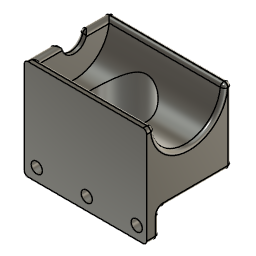
camera mount v2 (Autodesk Fusion 360 design; units mm, degrees)
Autodesk Fusion 360 part; units mm, degrees
sketch "Sketch1" plane through (0, 0, 0) normal (0, 0, 1) x (1, 0, 0)
  line L0 (0, 0) -> (49, 0)
  line L1 (49, 0) -> (49, 34)
  line L2 (49, 34) -> (0, 34)
  line L3 (0, 34) -> (0, 0)
  dimension "d1" = 49
  dimension "d2" = 34
  constraint horizontal L0
  constraint vertical L1
  constraint horizontal L2
  constraint vertical L3
  constraint coincident L0.start L3.end
  measures "d1" distance of L0.start L0.end
  measures "d2" distance of L0.start L2.end
extrude "Extrude1" add sketch "Sketch1" along normal blind 30
sketch "Sketch2" plane through (49, 0, 0) normal (1, 0, 0) x (0, 1, 0)
  line L0 (0, 0) -> (34, 0)
  line L1 (34, 0) -> (34, 30)
  line L2 (34, 30) -> (0, 30)
  line L3 (0, 30) -> (0, 0)
  circle A0 centre (17, 30) radius 14
  dimension "d5" = 28
  constraint midpoint L2 A0.centre
  measures "d5" diameter of A0
extrude "Extrude2" cut sketch "Sketch2" against normal blind 46 contours L2 A0 picked at (19.9096, 26.3515)
sketch "Sketch3" plane through (0, 0, 0) normal (0, 0, 1) x (1, 0, 0)
  circle A0 centre (21, 17) radius 11
  dimension "d10" = 22
  measures "d10" diameter of A0
extrude "Extrude3" cut sketch "Sketch3" along normal blind 40
sketch "Sketch4" plane through (3, 0, 0) normal (1, 0, 0) x (0, 1, 0)
  line L0 (31, 30) -> (3, 30)
  arc A0 (3, 30) -> (31, 30) centre (17, 30) ccw
  circle A1 centre (17, 30) radius 5
  dimension "d13" = 10
  constraint concentric A0 A1
  measures "d13" diameter of A1
extrude "Extrude4" cut sketch "Sketch4" against normal blind 3 contours L0 A1 picked at (18.5016, 28.7801)
sketch "Sketch5" plane through (0, 0, 0) normal (0, 0, -1) x (1, 0, 0)
  circle A0 centre (21, -17) radius 11
  line L0 (0, 0) -> (0, -34)
  line L1 (0, -34) -> (49, -34)
  line L2 (49, -34) -> (49, 0)
  line L3 (49, 0) -> (0, 0)
  line L4 (49, 0) -> (0, 0)
  line L5 (0, 0) -> (0, -5)
  line L6 (0, -5) -> (49, -5)
  line L7 (49, -5) -> (49, 0)
  dimension "d16" = 49
  dimension "d17" = 5
  constraint horizontal L4
  constraint vertical L5
  constraint horizontal L6
  constraint vertical L7
  constraint coincident L2.end L3.start
  measures "d16" distance of L2.end L0.start
  measures "d17" distance of L2.end L6.end
extrude "Extrude5" add sketch "Sketch5" along normal blind 10 contours L0 L2 L3 L4 L5 L6 L7
sketch "Sketch6" plane through (0, 5, 0) normal (0, 1, 0) x (-1, 0, 0)
  line L0 (0, 0) -> (-49, 0)
  line L1 (-49, 0) -> (-49, -10)
  line L2 (-49, -10) -> (0, -10)
  line L3 (0, -10) -> (0, 0)
  circle A0 centre (-5, -5) radius 2.25
  circle A1 centre (-25, -5) radius 2.25
  circle A2 centre (-45, -5) radius 2.25
  dimension "d20" = 4.5
  dimension "d22" = 4.5
  dimension "d24" = 4.5
  measures "d20" diameter of A0
  measures "d22" diameter of A1
  measures "d24" diameter of A2
extrude "Extrude6" cut sketch "Sketch6" against normal blind 5 contours A0 | A1 | A2
fillet "Fillet1" radius 1.5 25 edges at (49, 2.5, -10) (24.5, 5, -10) (49, 5, -5) (49, 19.5, 0) (24.5, 34, 0) (49, 34, 15) (24.5, 5, 0) (0, 19.5, 0) (0, 5, -5) (0, 2.5, -10) (0, 34, 15) (24.5, 34, 30) (0, 28, 30) (0, 17, 25) (0, 6, 30) (3, 7.5, 30) (1.5, 12, 30) (1.5, 22, 30) (3, 26.5, 30) (26, 31, 30) (49, 32.5, 30) (49, 17, 16) (49, 1.5, 30) (26, 3, 30) (10.7444, 13.0222, 0)
sketch "Sketch7" plane through (0, 0, 0) normal (0, 0, 1) x (1, 0, 0)
